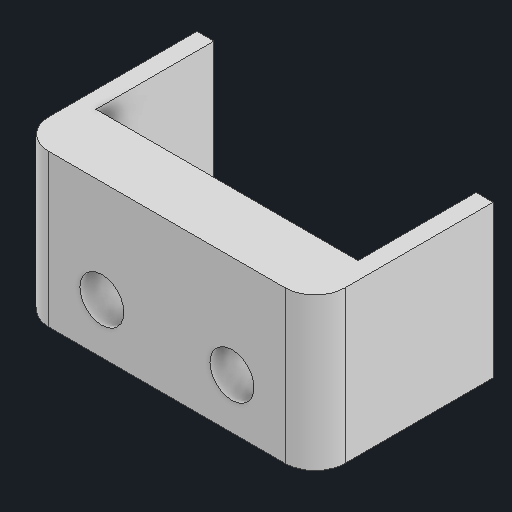
# Autodesk Inventor part: podkladka_switch
Saved by Autodesk Inventor 2023.4 (Build 274418000, 418)
## iProperties
Created: 2024-08-05
Part Number: podkladka_switch
Material: Generic
Document SubType Name: Modeling
Designer: komputer
Density: 1 g/cm^3
Appearance: Default
Author: komputer
Autodesk Inventor part; units mm, degrees
ref_plane "YZ Plane" through (0, 0, 0) normal (1, 0, 0) x (0, 1, 0)
ref_plane "XZ Plane" through (0, 0, 0) normal (0, 1, 0) x (-1, 0, 0)
sketch "Sketch1" plane through (0, 0, 0) normal (0, 0, 1) x (1, 0, 0)
  circle A0 centre (-3.25, -2.15) radius 1 projected
  circle A1 centre (3.25, -2.15) radius 1 projected
  circle A2 centre (-3.25, -2.15) radius 1.1
  circle A3 centre (3.25, -2.15) radius 1.1
  line L0 (-6.45, -0.55) -> (-6.45, -2.95) projected
  line L1 (6.45, -2.95) -> (6.45, -0.55) projected
  line L2 (-7.5, 2.95) -> (-10.5, 2.95) projected
  line L3 (10.5, 2.95) -> (7.5, 2.95) projected
  line L4 (-7.5, 2.95) -> (7.5, 2.95) projected
  line L5 (-6.45, 2.95) -> (-6.45, -0.55) projected
  line L6 (6.45, -0.55) -> (6.45, 2.95) projected
  line L7 (7.5, 2.95) -> (7.5, -8.05) projected
  line L8 (-7.5, 2.95) -> (-7.5, -6.5437) projected
  line L9 (-7.5, 2.95) -> (7.5, 2.95)
  line L10 (7.5, 2.95) -> (7.5, -4.65)
  line L11 (7.5, -4.65) -> (-7.5, -4.65)
  line L12 (-7.5, -4.65) -> (-7.5, 2.95)
  line L13 (-7.4, -4.65) -> (-7.4, 2.95)
  line L14 (7.4, -4.65) -> (7.4, 2.95)
  point P0 (0, 0)
  point P1 (-7.4, 2.95)
  point P2 (7.4, 2.95)
  dimension "d0" = 0.1
  dimension "d1" = 0.1
  dimension "d2" = 7.6
  dimension "d3" = 0.1
  dimension "d4" = 0.1
  constraints: 12 end point, 5 point on line, 4 parallel, 2 centre point, 2 perpendicular, 1 horizontal
  measures "d0" radial gap between concentric circles of A0 A2
  measures "d1" radial gap between concentric circles of A1 A3
  measures "d2" distance between parallel lines of L11 L9
  measures "d3" distance between parallel lines of L8 L13
  measures "d4" distance between parallel lines of L10 L14
extrude "Extrusion1" add sketch "Sketch1" along normal blind 3 contours L4 L14 L11 L13
sketch "Sketch2" plane through (0, 0, 0) normal (0, 0, -1) x (-1, 0, 0)
  line L0 (-6.45, -0.55) -> (-6.45, 2.95) projected
  line L1 (-7.4, -4.65) -> (-7.4, 2.95) projected
  line L2 (6.45, 2.95) -> (6.45, -0.55) projected
  line L3 (7.4, 2.95) -> (7.4, -4.65) projected
  line L4 (-6.55, -0.55) -> (-6.55, 2.95)
  line L5 (6.55, 2.95) -> (6.55, -0.55)
  line L6 (-7.4, 2.95) -> (7.4, 2.95) projected
  line L7 (7.4, -4.65) -> (-7.4, -4.65) projected
  line L8 (-7.4, 2.95) -> (-6.55, 2.95)
  line L9 (-6.55, 2.95) -> (-6.55, -4.65)
  line L10 (-6.55, -4.65) -> (-7.4, -4.65)
  line L11 (-7.4, -4.65) -> (-7.4, 2.95)
  line L12 (6.55, 2.95) -> (7.4, 2.95)
  line L13 (7.4, 2.95) -> (7.4, -4.65)
  line L14 (7.4, -4.65) -> (6.55, -4.65)
  line L15 (6.55, -4.65) -> (6.55, 2.95)
  point P0 (0, 0)
  point P1 (6.55, -0.55)
  dimension "d7" = 0.1
  dimension "d8" = 0.1
  constraints: 20 end point, 6 parallel, 2 horizontal, 2 perpendicular, 1 collinear, 1 point on line
  measures "d7" distance between parallel lines of L0 L4
  measures "d8" distance between parallel lines of L2 L5
ref_plane "Work Plane1" through (-15.5277, -15.5154, -5.9) normal (0, 0, 1) x (1, 0, 0)
extrude "Extrusion2" add sketch "Sketch2" along normal up to surface (5.9 mm away) contours L1 L6 L4 L9 L7 | L15 L5 L6 L3 L7
fillet "Fillet1" radius 1.5 2 edges at (7.4, -0.85, 3) (-7.4, -0.85, 3)
body "Solid1"
